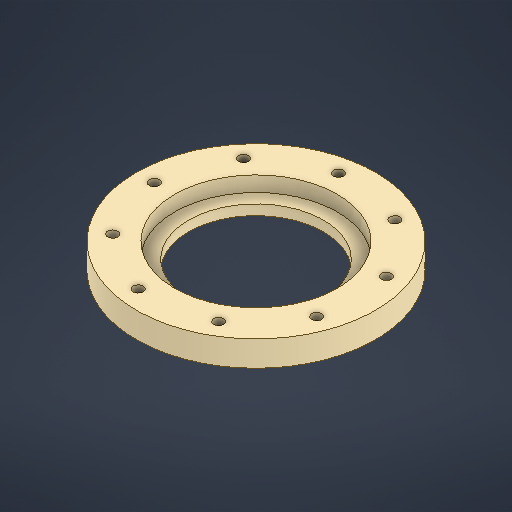
# Autodesk Inventor part: GFK_Ring_oben
Saved by Autodesk Inventor 2027 (Build 310192060, 192F)
## iProperties
Created: 2016-02-20
Part Number: GFK_Ring_oben
Material: Default New Material
Document SubType Name: Modeling
Designer: Halle20
Density: 1 g/cm^3
Appearance: Generic
Author: Halle20
Autodesk Inventor part; units mm, degrees
ref_plane "YZ Plane" through (0, 0, 0) normal (1, 0, 0) x (0, 1, 0)
ref_plane "XZ Plane" through (0, 0, 0) normal (0, 1, 0) x (-1, 0, 0)
ref_plane "XY Plane" through (0, 0, 0) normal (0, 0, 1) x (1, 0, 0)
sketch "Sketch9" plane through (0, 0, 0) normal (0, 1, 0) x (-1, 0, 0)
  circle A0 centre (0, 0) radius 32
  circle A1 centre (0, 0) radius 47
  circle A2 centre (0, 0) radius 26.5
  dimension "d54" = 64
  dimension "d55" = 94
  dimension "d56" = 53
  constraints: 3 centre point, 3 coincident
  measures "d54" diameter of A0
  measures "d55" diameter of A1
  measures "d56" diameter of A2
extrude "Extrusion8" add sketch "Sketch9" against normal blind 4 contours A0
extrude "Extrusion9" add sketch "Sketch9" against normal blind 10 contours A1
sketch "Sketch10" plane through (0, 0, 0) normal (0, 1, 0) x (1, 0, 0)
  circle A0 centre (0, 0) radius 40
  point P0 (-40, 0)
  point P1 (-30.6418, -25.7115)
  point P2 (-6.9459, -39.3923)
  point P3 (20, -34.641)
  point P4 (37.5877, -13.6808)
  point P5 (37.5877, 13.6808)
  point P6 (20, 34.641)
  point P7 (-6.9459, 39.3923)
  point P8 (-30.6418, 25.7115)
  dimension "d61" = 80
  dimension "d64" = 360
  constraints: 1 coincident, 1 horizontal alignment, 12 other
hole "Hole1" at (-40, 0, 0) at (-30.6418, 0, 25.7115) at (-6.9459, 0, 39.3923) at (20, 0, 34.641) at (37.5877, 0, 13.6808) at (37.5877, 0, -13.6808) at (20, 0, -34.641) at (-6.9459, 0, -39.3923) at (-30.6418, 0, -25.7115) direction (0, -1, 0) diameter 8 depth 5
hole "Hole2" at (-30.6418, 0, -25.7115) at (-6.9459, 0, -39.3923) at (20, 0, -34.641) at (37.5877, 0, -13.6808) at (37.5877, 0, 13.6808) at (-40, 0, 0) at (20, 0, 34.641) at (-6.9459, 0, 39.3923) at (-30.6418, 0, 25.7115) direction (0, -1, 0) diameter 4 depth 10
body "Solid2"
